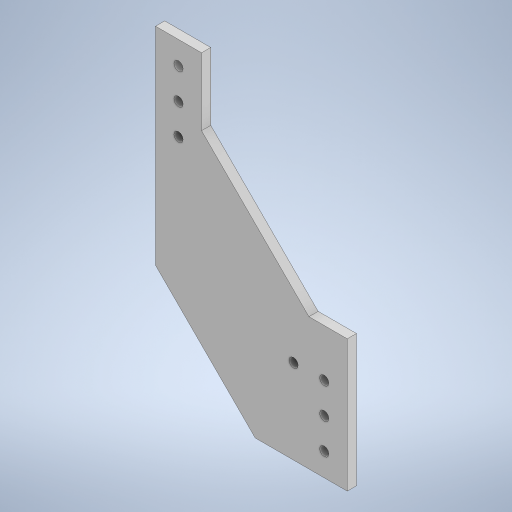
# Autodesk Inventor part: Plate_standard
Saved by Autodesk Inventor 2023 (Build 270158000, 158)
## iProperties
Created: 2024-02-04
Part Number: Plate_standard
Material: Generic
Document SubType Name: Modeling
Designer: victo
Density: 1 g/cm^3
Appearance: Default
Author: victo
Autodesk Inventor part; units mm, degrees
ref_plane "YZ Plane" through (0, 0, 0) normal (1, 0, 0) x (0, 1, 0)
ref_plane "XZ Plane" through (0, 0, 0) normal (0, 1, 0) x (-1, 0, 0)
ref_plane "XY Plane" through (0, 0, 0) normal (0, 0, 1) x (1, 0, 0)
sketch "Sketch1" plane through (0, 0, 0) normal (0, 0, 1) x (1, 0, 0)
  line L0 (0, 0) -> (-62.5, 0)
  line L1 (-62.5, 0) -> (-62.5, 100)
  line L2 (-62.5, 100) -> (0, 100)
  line L3 (0, 100) -> (0, 0)
  circle A0 centre (-7.5, 7.5) radius 1.5
  circle A1 centre (-7.5, 17.5) radius 1.5
  circle A2 centre (-7.5, 27.5) radius 1.5
  circle A3 centre (-17.5, 27.5) radius 1.5
  circle A4 centre (-55, 92.5) radius 1.5
  circle A5 centre (-55, 82.5) radius 1.5
  circle A6 centre (-55, 72.5) radius 1.5
  line L4 (0, 43) -> (-12.5, 43)
  line L5 (-12.5, 43) -> (-47.5, 78)
  line L6 (-47.5, 78) -> (-47.5, 100)
  line L7 (-30, 0) -> (-62.5, 32.5)
  dimension "d0" = 100
  dimension "d1" = 62.5
  dimension "d2" = 3
  dimension "d3" = 3
  dimension "d4" = 3
  dimension "d5" = 3
  dimension "d6" = 3
  dimension "d7" = 3
  dimension "d8" = 3
  dimension "d9" = 7.5
  dimension "d10" = 7.5
  dimension "d11" = 7.5
  dimension "d12" = 7.5
  dimension "d13" = 10
  dimension "d14" = 10
  dimension "d15" = 7.5
  dimension "d16" = 7.5
  dimension "d17" = 7.5
  dimension "d18" = 7.5
  dimension "d19" = 10
  dimension "d20" = 10
  dimension "d21" = 10
  dimension "d22" = 10
  dimension "d23" = 12.5
  dimension "d24" = 135
  dimension "d25" = 135
  dimension "d26" = 32.5
  dimension "d27" = 43
  dimension "d28" = 15
  constraints: 16 end point, 7 centre point, 4 point on line, 2 horizontal, 2 parallel, 2 perpendicular
  measures "d0" distance of L0.end L1.end
  measures "d1" distance between parallel lines of L3 L1
  measures "d2" diameter of A0
  measures "d3" diameter of A1
  measures "d4" diameter of A2
  measures "d5" diameter of A3
  measures "d6" diameter of A4
  measures "d7" diameter of A5
  measures "d8" diameter of A6
  measures "d9" distance from line of L2 A4.centre
  measures "d10" distance from line of L1 A4.centre
  measures "d11" distance from line of L1 A5.centre
  measures "d12" distance from line of L1 A6.centre
  measures "d13" distance of A4.centre A5.centre
  measures "d14" distance of A5.centre A6.centre
  measures "d15" distance from line of L3 A0.centre
  measures "d16" distance from line of L0 A0.centre
  measures "d17" distance from line of L3 A1.centre
  measures "d18" distance from line of L3 A2.centre
  measures "d19" distance of A1.centre A0.centre
  measures "d20" distance of A2.centre A1.centre
  measures "d21" distance of A3.centre A2.centre
  measures "d22" horizontal distance of A1.centre A3.centre
  measures "d23" distance of L4.start L4.end
  measures "d24" angle of L4 L5
  measures "d25" angle of L0 L7
  measures "d26" distance of L0.end L7.start
  measures "d27" distance between parallel lines of L0 L4
  measures "d28" distance between parallel lines of L1 L6
extrude "Extrusion1" add sketch "Sketch1" along normal blind 3 contours L0 L7 L1 L2 L6 L5 L4 L3
equation "\"d10\" = d9"
equation "\"d11\" = d9"
equation "\"d12\" = d11"
equation "\"d14\" = d13"
equation "\"d17\" = d15"
equation "\"d18\" = d15"
equation "\"d20\" = d19"
equation "\"d21\" = d19"
equation "\"d22\" = d19"
equation "\"d25\" = d24"
body "Solid1"
